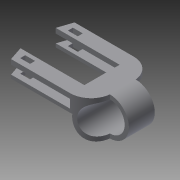
# Autodesk Inventor part: soporte camara
Saved by Autodesk Inventor 2013 (Build 170138000, 138)
## iProperties
Created: 2013-04-15
Part Number: soporte camara
Material: Generic
Document SubType Name: Modeling
Designer: Sebastian Saez
Density: 1 g/cm^3
Author: Sebastian Saez
Autodesk Inventor part; units mm, degrees
ref_plane "YZ Plane" through (0, 0, 0) normal (1, 0, 0) x (0, 1, 0)
ref_plane "XZ Plane" through (0, 0, 0) normal (0, 1, 0) x (-1, 0, 0)
ref_plane "XY Plane" through (0, 0, 0) normal (0, 0, 1) x (1, 0, 0)
sketch "Sketch1" plane through (0, 0, 0) normal (0, 1, 0) x (-1, 0, 0)
  circle A0 centre (0, 0) radius 10.5
  arc A1 (0, 13.5) -> (13.4164, 1.5) centre (0, 0) ccw
  line L0 (0, 13.5) -> (60, 13.5)
  line L1 (60, 13.5) -> (60, 1.5)
  line L2 (60, 1.5) -> (13.4164, 1.5)
  dimension "d1" = 21
  dimension "d2" = 60
  dimension "d3" = 12
  dimension "d6" = 3
  constraints: 6 end point, 2 centre point, 2 coincident, 2 point on circle, 1 horizontal, 1 parallel, 1 perpendicular, 1 tangent
  measures "d1" diameter of A0
  measures "d2" distance of L0.start L0.end
  measures "d3" distance of L0.end L1.end
  measures "d6" radial gap between concentric circles of A1 A0
extrude "Extrusion1" add sketch "Sketch1" along normal blind 45
sketch "Sketch2" plane through (-60, 0, 13.5) normal (0, 0, 1) x (1, 0, 0)
  line L0 (0, 45) -> (60, 45) projected
  line L1 (0, 35) -> (3.306, 45)
  line L2 (51.1457, 45) -> (3.306, 45)
  line L3 (0, 35) -> (45.2583, 35)
  line L4 (0, 22.5) -> (103.0931, 22.5) construction
  line L5 (0, 0) -> (60, 0)
  line L6 (0, 10) -> (3.306, 0)
  line L7 (0, 10) -> (45.2583, 10)
  line L8 (45.2583, 35) -> (45.2583, 10)
  line L9 (0, 35) -> (0, 10)
  line L10 (60, 0) -> (60, 45) projected
  line L11 (0, 10) -> (0, 0)
  line L12 (0, 0) -> (60, 0) projected
  line L13 (0, 45) -> (0, 35)
  line L14 (3.306, 45) -> (0, 45)
  constraints: 24 end point, 4 point on line, 3 parallel, 3 symmetric about line, 2 collinear, 2 perpendicular
extrude "Extrusion2" cut sketch "Sketch2" against normal blind 12 contours L0 L1 L13 | L3 L8 L7 L9 | L6 L5 L11
sketch "Sketch3" plane through (0, 45, 0) normal (0, 1, 0) x (1, 0, 0)
  line L0 (-60, -1.5) -> (-60, -13.5) projected
  line L1 (-60, -4) -> (-14.8943, -4)
  line L2 (-14.8943, -4) -> (-14.8943, -10)
  line L3 (-14.8943, -10) -> (-60, -10)
  line L4 (-60, -4) -> (-60, -10)
  constraints: 8 end point, 3 perpendicular, 2 point on line, 1 parallel
extrude "Extrusion3" cut sketch "Sketch3" against normal blind 45
sketch "Sketch4" plane through (0, 0, 13.5) normal (0, 0, 1) x (1, 0, 0)
  line L0 (-56.694, 0) -> (0, 0) projected
  line L1 (0, 0) -> (0, 45) projected
  line L2 (-56.694, 45) -> (0, 45) projected
  arc A0 (0, 31.6668) -> (-14.7825, 45) centre (-14.7825, 30.1387) ccw
  line L3 (0, 31.6668) -> (14.4337, 31.6668)
  line L4 (-19.4308, 22.5) -> (16.7273, 22.5) construction
  line L5 (14.4337, 31.6668) -> (14.4337, 22.5)
  line L6 (0, 13.3332) -> (14.4337, 13.3332)
  line L7 (14.4337, 13.3332) -> (14.4337, 22.5)
  arc A1 (-14.7825, 0) -> (0, 13.3332) centre (-14.7825, 14.8613) ccw
  line L8 (-14.7825, 45) -> (14.4337, 45)
  line L9 (14.4337, 45) -> (14.4337, 31.6668)
  line L10 (14.4337, 13.3332) -> (14.4337, 0)
  line L11 (14.4337, 0) -> (-14.7825, 0)
  constraints: 18 end point, 5 point on circle, 4 point on line, 4 symmetric about line, 2 centre point, 2 collinear, 2 parallel, 2 perpendicular, 2 tangent, 1 other
extrude "Extrusion4" cut sketch "Sketch4" against normal blind 45 contours A1 L1 L0 | L1 L6 L10 L11 | A0 L2 L1 | L1 L8 L9 L3
sketch "Sketch5" plane through (-60, 35, 13.5) normal (0, 0, 1) x (1, 0, 0)
  line L0 (45.2583, 0) -> (45.2583, -25) projected
  line L1 (12.9797, 6.1743) -> (5.9797, 6.1743)
  line L2 (5.9797, 6.1743) -> (5.9797, 2.6291)
  line L3 (5.9797, 2.6291) -> (12.9797, 2.6291)
  line L4 (12.9797, 2.6291) -> (12.9797, 6.1743)
  line L5 (45.2583, -12.5) -> (-11.096, -12.5) construction
  line L6 (12.9797, -31.1743) -> (5.9797, -31.1743)
  line L7 (5.9797, -31.1743) -> (5.9797, -27.6291)
  line L8 (5.9797, -27.6291) -> (12.9797, -27.6291)
  line L9 (12.9797, -27.6291) -> (12.9797, -31.1743)
  point P0 (60, -35)
  dimension "d16" = 7
  constraints: 18 end point, 4 symmetric about line, 2 parallel, 2 perpendicular, 1 horizontal, 1 midpoint
  measures "d16" distance of L3.end L2.end
extrude "Extrusion5" cut sketch "Sketch5" against normal blind 15
body "Solid1"
